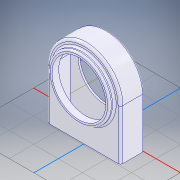
# Autodesk Inventor part: B6015L12F NF1
Saved by Autodesk Inventor 2022 (Build 260153000, 153)
## iProperties
Created: 2023-04-23
Part Number: B6015L12F NF1
Material: Стекло
Document SubType Name: Modeling
Designer: Иван Петров
Density: 2.18 g/cm^3
Appearance: Белая холодная
Author: Иван Петров
Autodesk Inventor part; units mm, degrees
ref_plane "YZ Plane" through (0, 0, 0) normal (1, 0, 0) x (0, 1, 0)
ref_plane "XZ Plane" through (0, 0, 0) normal (0, 1, 0) x (-1, 0, 0)
sketch "Эскиз1" plane through (0, 0, 0) normal (0, 0, 1) x (1, 0, 0)
  line L0 (-30, -35.5) -> (30, -35.5)
  line L1 (30, -35.5) -> (30, 35.5)
  line L2 (30, 35.5) -> (-30, 35.5)
  line L3 (-30, 35.5) -> (-30, -35.5)
  line L4 (-30, -35.5) -> (30, 35.5) construction
  line L5 (30, -35.5) -> (-30, 35.5) construction
  point P0 (0, 0)
  dimension "d0" = 60
  dimension "d1" = 71
  constraints: 12 end point, 2 midpoint, 2 parallel, 1 horizontal, 1 perpendicular
  measures "d0" distance of L2.end L1.end
  measures "d1" distance of L1.end L0.end
extrude "Выдавливание1" add sketch "Эскиз1" along normal blind 19
sketch "Эскиз2" plane through (0, 0, 19) normal (0, 0, 1) x (1, 0, 0)
  circle A0 centre (0, 5.5) radius 22 construction
  circle A1 centre (0, 5.5) radius 30
  line L0 (30, 35.5) -> (-30, 35.5) projected
  line L1 (-30, 35.5) -> (-30, -35.5) projected
  line L2 (30, -35.5) -> (30, 35.5) projected
  point P0 (0, 0)
  point P1 (30, 5.5)
  point P2 (0, 35.5)
  point P3 (-30, 5.5)
  dimension "d4" = 44
  dimension "d5" = 60
  dimension "d6" = 8
  constraints: 2 centre point, 1 coincident, 1 vertical alignment
  measures "d4" diameter of A0
  measures "d5" diameter of A1
  measures "d6" distance edge to line of A0 L0
extrude "Выдавливание2" cut sketch "Эскиз2" against normal through all contours A1 L0 L2 | A1 L1 L0
sketch "Эскиз3" plane through (0, 0, 19) normal (0, 0, 1) x (1, 0, 0)
  circle A0 centre (0, 5.5) radius 25
  arc A1 (30, 5.5) -> (-30, 5.5) centre (0, 5.5) ccw projected
  circle A2 centre (0, 5.5) radius 22
  point P0 (0, 0)
  dimension "d9" = 50
  dimension "d10" = 44
  constraints: 2 centre point, 1 coincident, 1 concentric
  measures "d9" diameter of A0
  measures "d10" diameter of A2
extrude "Выдавливание3" add sketch "Эскиз3" along normal blind 4
fillet "Сопряжение1" radius 1.5 2 edges at (-25, 5.5, 19) (-25, 5.5, 23)
sketch "Эскиз4" plane through (0, 5.5, 19) normal (0, 0, 1) x (1, 0, 0)
  circle A0 centre (0, 0) radius 22 projected
  point P0 (0, -5.5)
extrude "Выдавливание4" cut sketch "Эскиз4" against normal through all
sketch "Эскиз5" plane through (-30, -35.5, 0) normal (0, -1, 0) x (1, 0, 0)
  line L0 (1.5, 1.5) -> (58.5, 1.5)
  line L1 (58.5, 1.5) -> (58.5, 17.5)
  line L2 (58.5, 17.5) -> (1.5, 17.5)
  line L3 (1.5, 17.5) -> (1.5, 1.5)
  line L4 (60, 0) -> (60, 19) projected
  line L5 (0, 0) -> (60, 0) projected
  line L6 (0, 19) -> (60, 19) projected
  line L7 (0, 0) -> (0, 19) projected
  point P0 (30, 0)
  point P1 (30, 9.5)
  point P2 (30, 9.5)
  point P3 (60, 9.5)
  point P4 (30, 9.5)
  point P5 (30, 0)
  dimension "d16" = 1.5
  dimension "d17" = 1.5
  dimension "d18" = 1.5
  dimension "d19" = 1.5
  constraints: 8 end point, 2 midpoint, 2 parallel, 1 horizontal, 1 horizontal alignment, 1 perpendicular, 1 vertical alignment
  measures "d16" distance between parallel lines of L5 L0
  measures "d17" distance between parallel lines of L4 L1
  measures "d18" distance between parallel lines of L6 L2
  measures "d19" distance between parallel lines of L7 L3
ref_plane "РабПлоскость1" through (0, 5.5, 19) normal (0, -1, 0) x (0, 0, 1)
extrude "Выдавливание5" cut sketch "Эскиз5" against normal up to surface (41 mm away) contours L3 L2 L1 L0
sketch "Эскиз6" plane through (-28.5, 5.5, 17.5) normal (0, -1, 0) x (1, 0, 0)
  line L0 (6.5, 0) -> (6.5, -16) projected
  line L1 (0, 0) -> (6.5, 0) projected
  line L2 (0, -16) -> (0, 0) projected
  line L3 (6.5, -16) -> (0, -16) projected
  line L4 (28.5, -22.1) -> (28.5, 10.1) projected
  point P0 (28.5, -17.5)
revolve "Вращение1" cut sketch "Эскиз6" angle 180 about axis through (0, 5.5, 19) along (0, 0, -1)
fillet "Сопряжение2" radius 1 3 edges at (0, 35.5, 0) (30, -15, 0) (-30, -15, 0)
fillet "Сопряжение3" radius 2 3 edges at (0, 35.5, 19) (30, -15, 19) (-30, -15, 19)
equation "\"d17\" = d16"
equation "\"d18\" = d17"
equation "\"d19\" = d18"
